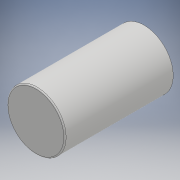
# Autodesk Inventor part: CanSatHousing
Saved by Autodesk Inventor 2018 (Build 220112000, 112)
## iProperties
Created: 2018-03-21
Part Number: CanSatHousing
Material: Generic
Document SubType Name: Modeling
Designer: boeingnut
Density: 1 g/cm^3
Appearance: Default
Author: boeingnut
Autodesk Inventor part; units mm, degrees
ref_plane "YZ Plane" through (0, 0, 0) normal (1, 0, 0) x (0, 1, 0)
ref_plane "XZ Plane" through (0, 0, 0) normal (0, 1, 0) x (-1, 0, 0)
ref_plane "XY Plane" through (0, 0, 0) normal (0, 0, 1) x (1, 0, 0)
sketch "Sketch1" plane through (0, 0, 0) normal (0, 1, 0) x (-1, 0, 0)
  circle A0 centre (0, 0) radius 25
  circle A1 centre (0, 0) radius 24
  dimension "d0" = 50
  dimension "d1" = 48
  constraints: 2 centre point, 2 coincident
  measures "d0" diameter of A0
  measures "d1" diameter of A1
extrude "Extrusion1" add sketch "Sketch1" along normal blind 90
sketch "Sketch2" plane through (0, 0, 0) normal (0, -1, 0) x (1, 0, 0)
  circle A0 centre (0, 0) radius 25 projected
extrude "Extrusion2" add sketch "Sketch2" along normal blind 3
fillet "Fillet1" radius 3 1 edges at (24, 0, 0)
fillet "Fillet2" radius 1 1 edges at (-25, -3, 0)
sketch "Sketch3" plane through (0, 90, 0) normal (0, 1, 0) x (1, 0, 0)
  circle A0 centre (0, 0) radius 24 projected
  line L0 (-26.5, -1) -> (-21.5, -1)
  line L1 (-21.5, -1) -> (-21.5, 1)
  line L2 (-21.5, 1) -> (-26.5, 1)
  line L3 (-26.5, 1) -> (-26.5, -1)
  line L4 (-26.5, -1) -> (-21.5, 1) construction
  line L5 (-21.5, -1) -> (-26.5, 1) construction
  line L6 (1, -26.5) -> (1, -21.5)
  line L7 (1, -21.5) -> (-1, -21.5)
  line L8 (-1, -21.5) -> (-1, -26.5)
  line L9 (-1, -26.5) -> (1, -26.5)
  line L10 (26.5, 1) -> (21.5, 1)
  line L11 (21.5, 1) -> (21.5, -1)
  line L12 (21.5, -1) -> (26.5, -1)
  line L13 (26.5, -1) -> (26.5, 1)
  line L14 (-1, 26.5) -> (-1, 21.5)
  line L15 (-1, 21.5) -> (1, 21.5)
  line L16 (1, 21.5) -> (1, 26.5)
  line L17 (1, 26.5) -> (-1, 26.5)
  arc A1 (1, 23.9792) -> (-1, 23.9792) centre (0, 0) ccw
  arc A2 (-23.9792, 1) -> (-23.9792, -1) centre (0, 0) ccw
  arc A3 (-1, -23.9792) -> (1, -23.9792) centre (0, 0) ccw
  arc A4 (23.9792, -1) -> (23.9792, 1) centre (0, 0) ccw
  point P0 (-24, 0)
  dimension "d8" = 5
  dimension "d9" = 2
  dimension "d12" = 360
  constraints: 36 end point, 8 point on circle, 8 point on line, 4 centre point, 2 midpoint, 2 parallel, 1 coincident, 1 horizontal, 1 horizontal alignment, 1 perpendicular, 34 other
  measures "d8" distance of L2.end L1.end
  measures "d9" distance of L1.end L0.end
extrude "Extrusion3" add sketch "Sketch3" against normal blind 92 contours A0 L12 L11 L10 | L16 L15 L14 A0 | A0 L8 L7 L6 | L2 L1 L0 A0
fillet "Fillet3" radius 1 8 edges at (21.5, 45.023, 1) (21.5, 45.023, -1) (1, 45.023, 21.5) (-1, 45.023, 21.5) (-21.5, 45.023, 1) (-21.5, 45.023, -1) (-1, 45.023, -21.5) (1, 45.023, -21.5)
fillet "Fillet4" radius 1 26 edges at (23.583, 1.5106, -1) (21.8177, 0.1171, -0.7314) (21.8177, 0.1171, 0.7314) (23.583, 1.5106, 1) (23.9792, 46.5, 1) (23.9792, 46.5, -1) (-1, 1.5106, 23.583) (-0.7314, 0.1171, 21.8177) (0.7314, 0.1171, 21.8177) (1, 1.5106, 23.583) (1, 46.5, 23.9792) (-1, 46.5, 23.9792) (-23.583, 1.5106, -1) (-21.5, 0.042, -0.0003) (-21.8177, 0.1171, -0.7314) (-21.5, 0.042, 0.0003) (-21.8177, 0.1171, 0.7314) (-23.583, 1.5106, 1) (-23.9792, 46.5, 1) (-23.9792, 46.5, -1) (-1, 1.5106, -23.583) (-0.7314, 0.1171, -21.8177) (0.7314, 0.1171, -21.8177) (1, 1.5106, -23.583) (1, 46.5, -23.9792) (-1, 46.5, -23.9792)
sketch "Sketch4" plane through (0, 90, 0) normal (0, 1, 0) x (1, 0, 0)
  circle A0 centre (0, 0) radius 24
  constraints: 1 centre point, 1 coincident
extrude "Extrusion4" cut sketch "Sketch4" against normal blind 5
body "Solid1"
